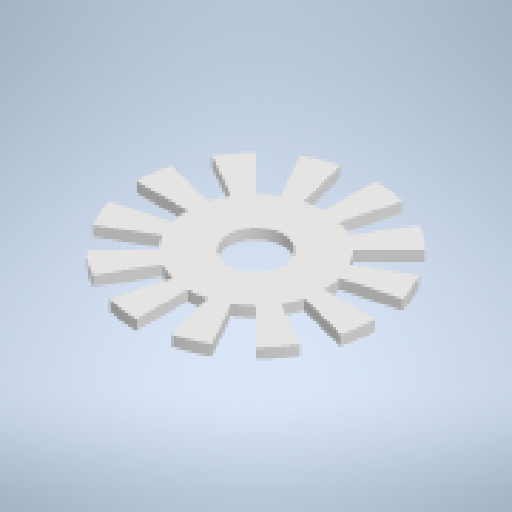
# Autodesk Inventor part: Encoder2
Saved by Autodesk Inventor 2023 (Build 270158000, 158)
## iProperties
Created: 2022-12-24
Part Number: Encoder2
Material: Genérico
Document SubType Name: Modeling
Designer: sergi
Density: 1 g/cm^3
Appearance: Valor por defecto
Author: sergi
Autodesk Inventor part; units mm, degrees
ref_plane "YZ Plane" through (0, 0, 0) normal (1, 0, 0) x (0, 1, 0)
ref_plane "XZ Plane" through (0, 0, 0) normal (0, 1, 0) x (-1, 0, 0)
ref_plane "XY Plane" through (0, 0, 0) normal (0, 0, 1) x (1, 0, 0)
sketch "Boceto1" plane through (0, 0, 0) normal (0, 1, 0) x (-1, 0, 0)
  line L0 (0, -10) -> (0, -17.5)
  arc A0 (0, -10) -> (2.5882, -9.6593) centre (0, 0) ccw
  line L1 (2.5882, -9.6593) -> (4.5293, -16.9037)
  line L2 (5, -8.6603) -> (8.75, -15.1554)
  arc A1 (5, -8.6603) -> (7.0711, -7.0711) centre (0, 0) ccw
  line L3 (7.0711, -7.0711) -> (12.3744, -12.3744)
  line L4 (8.6603, -5) -> (15.1554, -8.75)
  arc A2 (8.6603, -5) -> (9.6593, -2.5882) centre (0, 0) ccw
  line L5 (9.6593, -2.5882) -> (16.9037, -4.5293)
  line L6 (10, 0) -> (17.5, 0)
  arc A3 (10, 0) -> (9.6593, 2.5882) centre (0, 0) ccw
  line L7 (9.6593, 2.5882) -> (16.9037, 4.5293)
  line L8 (8.6603, 5) -> (15.1554, 8.75)
  arc A4 (8.6603, 5) -> (7.0711, 7.0711) centre (0, 0) ccw
  line L9 (7.0711, 7.0711) -> (12.3744, 12.3744)
  line L10 (5, 8.6603) -> (8.75, 15.1554)
  arc A5 (5, 8.6603) -> (2.5882, 9.6593) centre (0, 0) ccw
  line L11 (2.5882, 9.6593) -> (4.5293, 16.9037)
  line L12 (0, 10) -> (0, 17.5)
  arc A6 (0, 10) -> (-2.5882, 9.6593) centre (0, 0) ccw
  line L13 (-2.5882, 9.6593) -> (-4.5293, 16.9037)
  line L14 (-5, 8.6603) -> (-8.75, 15.1554)
  arc A7 (-5, 8.6603) -> (-7.0711, 7.0711) centre (0, 0) ccw
  line L15 (-7.0711, 7.0711) -> (-12.3744, 12.3744)
  line L16 (-8.6603, 5) -> (-15.1554, 8.75)
  arc A8 (-8.6603, 5) -> (-9.6593, 2.5882) centre (0, 0) ccw
  line L17 (-9.6593, 2.5882) -> (-16.9037, 4.5293)
  line L18 (-10, 0) -> (-17.5, 0)
  arc A9 (-10, 0) -> (-9.6593, -2.5882) centre (0, 0) ccw
  line L19 (-9.6593, -2.5882) -> (-16.9037, -4.5293)
  line L20 (-8.6603, -5) -> (-15.1554, -8.75)
  arc A10 (-8.6603, -5) -> (-7.0711, -7.0711) centre (0, 0) ccw
  line L21 (-7.0711, -7.0711) -> (-12.3744, -12.3744)
  line L22 (-5, -8.6603) -> (-8.75, -15.1554)
  arc A11 (-5, -8.6603) -> (-2.5882, -9.6593) centre (0, 0) ccw
  line L23 (-2.5882, -9.6593) -> (-4.5293, -16.9037)
  arc A12 (12.3744, 12.3744) -> (8.75, 15.1554) centre (0, 0) ccw
  arc A13 (16.9037, 4.5293) -> (15.1554, 8.75) centre (0, 0) ccw
  arc A14 (16.9037, -4.5293) -> (17.5, 0) centre (0, 0) ccw
  arc A15 (12.3744, -12.3744) -> (15.1554, -8.75) centre (0, 0) ccw
  arc A16 (4.5293, -16.9037) -> (8.75, -15.1554) centre (0, 0) ccw
  arc A17 (-4.5293, -16.9037) -> (0, -17.5) centre (0, 0) ccw
  arc A18 (-12.3744, -12.3744) -> (-8.75, -15.1554) centre (0, 0) ccw
  arc A19 (-16.9037, -4.5293) -> (-15.1554, -8.75) centre (0, 0) ccw
  arc A20 (-16.9037, 4.5293) -> (-17.5, 0) centre (0, 0) ccw
  arc A21 (-12.3744, 12.3744) -> (-15.1554, 8.75) centre (0, 0) ccw
  arc A22 (4.5293, 16.9037) -> (0, 17.5) centre (0, 0) ccw
  arc A23 (-4.5293, 16.9037) -> (-8.75, 15.1554) centre (0, 0) ccw
  line L24 (5.1962, 3) -> (7.1962, 3)
  line L25 (7.1962, 3) -> (7.1962, -3)
  line L26 (7.1962, -3) -> (5.1962, -3)
  line L27 (-5.1962, -3) -> (-7.1962, -3)
  line L28 (-7.1962, -3) -> (-7.1962, 3)
  line L29 (-7.1962, 3) -> (-5.1962, 3)
  arc A24 (5.1962, 3) -> (-5.1962, 3) centre (0, 0) ccw
  arc A25 (-5.1962, -3) -> (5.1962, -3) centre (0, 0) ccw
  dimension "d6" = 360
  dimension "d11" = 2
  dimension "d12" = 6
  dimension "d13" = 2
  dimension "d14" = 6
  constraints: 60 end point, 52 point on circle, 26 centre point, 2 coincident, 2 perpendicular, 2 point on line, 1 vertical, 97 other
  measures "d11" distance of L24.start L24.end
  measures "d12" distance of L24.end L25.end
  measures "d13" distance of L27.start L27.end
  measures "d14" distance of L27.end L28.end
extrude "Extrusión1" add sketch "Boceto1" along normal blind 1.5 contours L0 A17 L23 A11 L22 A18 L21 A10 L20 A19 L19 A9 L18 A20 L17 A8 L16 A21 L15 A7 L14 A23 L13 A6 L12 A22 L11 A5 L10 A12 L9 A4 L8 A13 L7 A3 L6 A14 L5 A2 L4 A15 L3 A1 L2 A16 L1 A0 | L24 L25 L26 A25 L27 L28 L29 A24
sketch "Boceto2" plane through (0, 0, 0) normal (0, -1, 0) x (1, 0, 0)
  arc A0 (-9.6593, -2.5882) -> (-8.6603, -5) centre (0, 0) ccw projected
  constraints: 1 coincident
hole "Agujero1" at (0, 0, 0) direction (0, 1, 0) diameter 8 depth 8 tip angle 118
